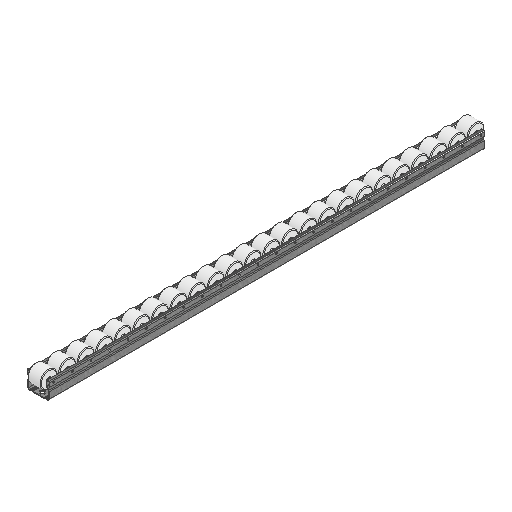
# Autodesk Inventor part: Trilho Roletado Flow Rack 40
Saved by Autodesk Inventor 2026.1 (Build 301233000, 233)
## iProperties
Company: Elgin
Created: 2024-05-28
Part Number: Trilho Roletado Flow Rack 40
Material: Genérico
Document SubType Name: Modeling
Designer: Willian Pinheiro
Density: 1 g/cm^3
Appearance: Padrão
Mass: 662.162 g
Surface Area: 3287.54 cm^2
Volume: 662.162 cm^3
Checked By: Antonio Lucas
Engr Approved By: Antonio Lucas
Description: Trilho Roletado Flow Rack 40
Mfg Approved By: Anderson Oliveira
Dimensões: 800 mm
Total: 8
Author: Willian Pinheiro
Title: Ceteva
Revision Number: 00
Autodesk Inventor part; units mm, degrees
ref_plane "YZ Plane" through (0, 0, 0) normal (1, 0, 0) x (0, 1, 0)
sketch "trilho roletado 40" plane through (0, 0, 0) normal (0, 0, 1) x (1, 0, 0)
  line L0 (54.5, 1.2) -> (54.5, -1.2)
  line L1 (54.5, -1.2) -> (54, -1.7)
  line L2 (54, -1.7) -> (16, -1.7)
  line L3 (49, -1.7) -> (49, -4)
  line L4 (49, -4) -> (47.5, -4)
  line L5 (47.5, -4) -> (47.5, -14.6092)
  arc A0 (46.1065, -16.1054) -> (47.5, -14.6092) centre (46, -14.6092) ccw
  arc A1 (23.8935, -16.1054) -> (46.1065, -16.1054) centre (35, 140) ccw
  arc A2 (22.5, -14.6092) -> (23.8935, -16.1054) centre (24, -14.6092) ccw
  line L6 (22.5, -14.6092) -> (22.5, -4)
  line L7 (22.5, -4) -> (21, -4)
  line L8 (21, -4) -> (21, -1.7)
  line L9 (16, -1.7) -> (15.5, -1.2)
  line L10 (15.5, -1.2) -> (15.5, 1.2)
  line L11 (15.5, 1.2) -> (16, 1.7)
  line L12 (21, 1.7) -> (21, 4)
  line L13 (21, 4) -> (22.5, 4)
  line L14 (22.5, 4) -> (22.5, 14.6092)
  arc A3 (23.8935, 16.1054) -> (22.5, 14.6092) centre (24, 14.6092) ccw
  arc A4 (46.1065, 16.1054) -> (23.8935, 16.1054) centre (35, -140) ccw
  arc A5 (47.5, 14.6092) -> (46.1065, 16.1054) centre (46, 14.6092) ccw
  line L15 (47.5, 14.6092) -> (47.5, 4)
  line L16 (47.5, 4) -> (49, 4)
  line L17 (49, 4) -> (49, 1.7)
  line L18 (16, 1.7) -> (54, 1.7)
  line L19 (54, 1.7) -> (54.5, 1.2)
  line L20 (13.5, -1.7865) -> (15, -1.7865)
  line L21 (15, -1.7865) -> (15, -4.5365)
  line L22 (15, -4.5365) -> (13.5, -4.5365)
  line L23 (13.5, -4.5365) -> (13.5, -1.7865)
  line L24 (20.5, 1.7135) -> (19, 1.7135)
  line L25 (19, 1.7135) -> (19, 3)
  line L26 (19, 3) -> (15, 3)
  line L27 (15, 3) -> (15, 1.7135)
  line L28 (15, 1.7135) -> (13.5, 1.7135)
  line L29 (13.5, 1.7135) -> (13.5, 3)
  arc A6 (15, 4.5) -> (13.5, 3) centre (15, 3) ccw
  line L30 (15, 4.5) -> (19, 4.5)
  arc A7 (20.5, 3) -> (19, 4.5) centre (19, 3) ccw
  line L31 (20.5, 3) -> (20.5, 1.7135)
  line L32 (56.5, 1.7135) -> (55, 1.7135)
  line L33 (55, 1.7135) -> (55, 3)
  line L34 (55, 3) -> (51, 3)
  line L35 (51, 3) -> (51, 1.7135)
  line L36 (51, 1.7135) -> (49.5, 1.7135)
  line L37 (49.5, 1.7135) -> (49.5, 3)
  arc A8 (51, 4.5) -> (49.5, 3) centre (51, 3) ccw
  line L38 (51, 4.5) -> (55, 4.5)
  arc A9 (56.5, 3) -> (55, 4.5) centre (55, 3) ccw
  line L39 (56.5, 3) -> (56.5, 1.7135)
  line L40 (55, -1.7865) -> (56.5, -1.7865)
  line L41 (56.5, -1.7865) -> (56.5, -4.5365)
  line L42 (56.5, -4.5365) -> (55, -4.5365)
  line L43 (55, -4.5365) -> (55, -1.7865)
  line L44 (40.75, -27) -> (45.3477, -27)
  arc A10 (45.3477, -27) -> (46.2081, -26.7287) centre (45.3477, -25.5) ccw
  line L45 (46.2081, -26.7287) -> (47.283, -25.9761)
  arc A11 (48.717, -25.9761) -> (47.283, -25.9761) centre (48, -27) ccw
  line L46 (48.717, -25.9761) -> (49.7919, -26.7287)
  arc A12 (49.7919, -26.7287) -> (50.6523, -27) centre (50.6523, -25.5) ccw
  line L47 (50.6523, -27) -> (51.5, -27)
  arc A13 (51.5, -27) -> (53.5, -25) centre (51.5, -25) ccw
  line L48 (53.5, -25) -> (53.5, -12.7967)
  arc A14 (53.5, -12.7967) -> (53.1047, -11.3083) centre (50.5, -12.7967) ccw
  line L49 (53.1047, -11.3083) -> (49.8953, -5.6917)
  arc A15 (49.5, -4.1668) -> (49.8953, -5.6917) centre (52.4998, -4.2029) ccw
  line L50 (49.5, -4.1668) -> (49.5, -1.7135)
  line L51 (49.5, -1.7135) -> (51, -1.7135)
  line L52 (51, -1.7135) -> (51, -4.1668)
  arc A16 (51, -4.1668) -> (51.1976, -4.9475) centre (52.4996, -4.2026) ccw
  line L53 (51.1976, -4.9475) -> (54.4071, -10.5641)
  arc A17 (55, -12.7967) -> (54.4071, -10.5641) centre (50.5, -12.7967) ccw
  line L54 (55, -12.7967) -> (55, -25)
  arc A18 (51.5, -28.5) -> (55, -25) centre (51.5, -25) ccw
  line L55 (51.5, -28.5) -> (50.6523, -28.5)
  arc A19 (48.9315, -27.9575) -> (50.6523, -28.5) centre (50.6523, -25.5) ccw
  line L56 (48.9315, -27.9575) -> (48, -27.3052)
  line L57 (48, -27.3052) -> (47.0685, -27.9575)
  arc A20 (45.3477, -28.5) -> (47.0685, -27.9575) centre (45.3477, -25.5) ccw
  line L58 (45.3477, -28.5) -> (40.75, -28.5)
  line L59 (29.25, -28.5) -> (24.6523, -28.5)
  arc A21 (22.9315, -27.9575) -> (24.6523, -28.5) centre (24.6523, -25.5) ccw
  line L60 (22.9315, -27.9575) -> (22, -27.3052)
  line L61 (22, -27.3052) -> (21.0685, -27.9575)
  arc A22 (19.3477, -28.5) -> (21.0685, -27.9575) centre (19.3477, -25.5) ccw
  line L62 (19.3477, -28.5) -> (18.5, -28.5)
  arc A23 (15, -25) -> (18.5, -28.5) centre (18.5, -25) ccw
  line L63 (15, -25) -> (15, -12.7967)
  arc A24 (15.5929, -10.5276) -> (15, -12.7967) centre (19.4999, -12.7605) ccw
  line L64 (15.5929, -10.5276) -> (18.8024, -4.911)
  arc A25 (18.8024, -4.911) -> (19, -4.1668) centre (17.5, -4.1668) ccw
  line L65 (19, -4.1668) -> (19, -1.7135)
  line L66 (19, -1.7135) -> (20.5, -1.7135)
  line L67 (20.5, -1.7135) -> (20.5, -4.2398)
  arc A26 (20.1047, -5.7282) -> (20.5, -4.2398) centre (17.5, -4.2398) ccw
  line L68 (20.1047, -5.7282) -> (16.8953, -11.3448)
  arc A27 (16.8953, -11.3448) -> (16.5, -12.7967) centre (19.4998, -12.8336) ccw
  line L69 (16.5, -12.7967) -> (16.5, -25)
  arc A28 (16.5, -25) -> (18.5, -27) centre (18.5, -25) ccw
  line L70 (18.5, -27) -> (19.3477, -27)
  arc A29 (19.3477, -27) -> (20.2081, -26.7287) centre (19.3477, -25.5) ccw
  line L71 (20.2081, -26.7287) -> (21.283, -25.9761)
  arc A30 (22.717, -25.9761) -> (21.283, -25.9761) centre (22, -27) ccw
  line L72 (22.717, -25.9761) -> (23.7919, -26.7287)
  arc A31 (23.7919, -26.7287) -> (24.6523, -27) centre (24.6523, -25.5) ccw
  line L73 (24.6523, -27) -> (29.25, -27)
  line L74 (29.25, -27) -> (29.25, -28.5)
  line L75 (40.75, -27) -> (40.75, -28.5)
  line L76 (29.25, -27) -> (40.75, -27)
  line L77 (40.75, -28.5) -> (29.25, -28.5)
  line L78 (13.5, 1.7135) -> (13.5, -1.7865)
  line L79 (15, 1.7135) -> (15, -1.7865)
  line L80 (19, 1.7135) -> (19, -1.7135)
  line L81 (20.5, -1.7135) -> (20.5, 1.7135)
  line L82 (49.5, 1.7135) -> (49.5, -1.7135)
  line L83 (51, 1.7135) -> (51, -1.7135)
  line L84 (55, 1.7135) -> (55, -1.7865)
  line L85 (56.5, 1.7135) -> (56.5, -1.7865)
  line L86 (35, -28.5) -> (35, -27) construction
  line L87 (54.5, 0) -> (15.5, 0)
  point P0 (35, 0)
  dimension "d40" = 1.5
  dimension "d41" = 1.5
  dimension "d42" = 33
  dimension "d43" = 1.5
  dimension "d44" = 1.5
  dimension "d45" = 1.5
  measures "d40" distance between parallel lines of L26 L30
  measures "d41" radius of A6
  measures "d42" distance between parallel lines of L59 L30
  measures "d43" distance between parallel lines of L27 L29
  measures "d44" distance between parallel lines of L31 L25
  measures "d45" distance between parallel lines of L59 L73
sketch "Sketch1" plane through (0, 0, 0) normal (0, 1, 0) x (-1, 0, 0)
  line L0 (30.5349, 0) -> (-30.5349, 0) construction
  line L1 (0, -167.5) -> (0, 224.5) construction
  line L2 (19.5, 29.7) -> (19.5, 27.3)
  line L3 (19.5, 27.3) -> (19, 26.8)
  line L4 (19, 26.8) -> (-19, 26.8)
  line L5 (14, 26.8) -> (14, 24.5)
  line L6 (14, 24.5) -> (12.5, 24.5)
  line L7 (12.5, 24.5) -> (12.5, 13.8908)
  arc A0 (11.1065, 12.3946) -> (12.5, 13.8908) centre (11, 13.8908) ccw
  arc A1 (-11.1065, 12.3946) -> (11.1065, 12.3946) centre (0, 168.5) ccw
  arc A2 (-12.5, 13.8908) -> (-11.1065, 12.3946) centre (-11, 13.8908) ccw
  line L8 (-12.5, 13.8908) -> (-12.5, 24.5)
  line L9 (-12.5, 24.5) -> (-14, 24.5)
  line L10 (-14, 24.5) -> (-14, 26.8)
  line L11 (-19, 26.8) -> (-19.5, 27.3)
  line L12 (-19.5, 27.3) -> (-19.5, 29.7)
  line L13 (-19.5, 29.7) -> (-19, 30.2)
  line L14 (-14, 30.2) -> (-14, 32.5)
  line L15 (-14, 32.5) -> (-12.5, 32.5)
  line L16 (-12.5, 32.5) -> (-12.5, 43.1092)
  arc A3 (-11.1065, 44.6054) -> (-12.5, 43.1092) centre (-11, 43.1092) ccw
  arc A4 (11.1065, 44.6054) -> (-11.1065, 44.6054) centre (0, -111.5) ccw
  arc A5 (12.5, 43.1092) -> (11.1065, 44.6054) centre (11, 43.1092) ccw
  line L17 (12.5, 43.1092) -> (12.5, 32.5)
  line L18 (12.5, 32.5) -> (14, 32.5)
  line L19 (14, 32.5) -> (14, 30.2)
  line L20 (-19, 30.2) -> (19, 30.2)
  line L21 (19, 30.2) -> (19.5, 29.7)
  line L22 (-21.5, 26.7135) -> (-20, 26.7135)
  line L23 (-20, 26.7135) -> (-20, 23.9635)
  line L24 (-20, 23.9635) -> (-21.5, 23.9635)
  line L25 (-21.5, 23.9635) -> (-21.5, 26.7135)
  line L26 (-14.5, 30.2135) -> (-16, 30.2135)
  line L27 (-16, 30.2135) -> (-16, 31.5)
  line L28 (-16, 31.5) -> (-20, 31.5)
  line L29 (-20, 31.5) -> (-20, 30.2135)
  line L30 (-20, 30.2135) -> (-21.5, 30.2135)
  line L31 (-21.5, 30.2135) -> (-21.5, 31.5)
  arc A6 (-20, 33) -> (-21.5, 31.5) centre (-20, 31.5) ccw
  line L32 (-20, 33) -> (-16, 33)
  arc A7 (-14.5, 31.5) -> (-16, 33) centre (-16, 31.5) ccw
  line L33 (-14.5, 31.5) -> (-14.5, 30.2135)
  line L34 (21.5, 30.2135) -> (20, 30.2135)
  line L35 (20, 30.2135) -> (20, 31.5)
  line L36 (20, 31.5) -> (16, 31.5)
  line L37 (16, 31.5) -> (16, 30.2135)
  line L38 (16, 30.2135) -> (14.5, 30.2135)
  line L39 (14.5, 30.2135) -> (14.5, 31.5)
  arc A8 (16, 33) -> (14.5, 31.5) centre (16, 31.5) ccw
  line L40 (16, 33) -> (20, 33)
  arc A9 (21.5, 31.5) -> (20, 33) centre (20, 31.5) ccw
  line L41 (21.5, 31.5) -> (21.5, 30.2135)
  line L42 (20, 26.7135) -> (21.5, 26.7135)
  line L43 (21.5, 26.7135) -> (21.5, 23.9635)
  line L44 (21.5, 23.9635) -> (20, 23.9635)
  line L45 (20, 23.9635) -> (20, 26.7135)
  line L46 (5.75, 1.5) -> (10.3477, 1.5)
  arc A10 (10.3477, 1.5) -> (11.2081, 1.7713) centre (10.3477, 3) ccw
  line L47 (11.2081, 1.7713) -> (12.283, 2.5239)
  arc A11 (13.717, 2.5239) -> (12.283, 2.5239) centre (13, 1.5) ccw
  line L48 (13.717, 2.5239) -> (14.7919, 1.7713)
  arc A12 (14.7919, 1.7713) -> (15.6523, 1.5) centre (15.6523, 3) ccw
  line L49 (15.6523, 1.5) -> (16.5, 1.5)
  arc A13 (16.5, 1.5) -> (18.5, 3.5) centre (16.5, 3.5) ccw
  line L50 (18.5, 3.5) -> (18.5, 15.7033)
  arc A14 (18.5, 15.7033) -> (18.1047, 17.1917) centre (15.5, 15.7033) ccw
  line L51 (18.1047, 17.1917) -> (14.8953, 22.8083)
  arc A15 (14.5, 24.3332) -> (14.8953, 22.8083) centre (17.4998, 24.2971) ccw
  line L52 (14.5, 24.3332) -> (14.5, 26.7865)
  line L53 (14.5, 26.7865) -> (16, 26.7865)
  line L54 (16, 26.7865) -> (16, 24.3332)
  arc A16 (16, 24.3332) -> (16.1976, 23.5525) centre (17.4996, 24.2974) ccw
  line L55 (16.1976, 23.5525) -> (19.4071, 17.9359)
  arc A17 (20, 15.7033) -> (19.4071, 17.9359) centre (15.5, 15.7033) ccw
  line L56 (20, 15.7033) -> (20, 3.5)
  arc A18 (16.5, 0) -> (20, 3.5) centre (16.5, 3.5) ccw
  line L57 (16.5, 0) -> (15.6523, 0)
  arc A19 (13.9315, 0.5425) -> (15.6523, 0) centre (15.6523, 3) ccw
  line L58 (13.9315, 0.5425) -> (13, 1.1948)
  line L59 (13, 1.1948) -> (12.0685, 0.5425)
  arc A20 (10.3477, 0) -> (12.0685, 0.5425) centre (10.3477, 3) ccw
  line L60 (10.3477, 0) -> (5.75, 0)
  line L61 (-5.75, 0) -> (-10.3477, 0)
  arc A21 (-12.0685, 0.5425) -> (-10.3477, 0) centre (-10.3477, 3) ccw
  line L62 (-12.0685, 0.5425) -> (-13, 1.1948)
  line L63 (-13, 1.1948) -> (-13.9315, 0.5425)
  arc A22 (-15.6523, 0) -> (-13.9315, 0.5425) centre (-15.6523, 3) ccw
  line L64 (-15.6523, 0) -> (-16.5, 0)
  arc A23 (-20, 3.5) -> (-16.5, 0) centre (-16.5, 3.5) ccw
  line L65 (-20, 3.5) -> (-20, 15.7033)
  arc A24 (-19.4071, 17.9724) -> (-20, 15.7033) centre (-15.5001, 15.7395) ccw
  line L66 (-19.4071, 17.9724) -> (-16.1976, 23.589)
  arc A25 (-16.1976, 23.589) -> (-16, 24.3332) centre (-17.5, 24.3332) ccw
  line L67 (-16, 24.3332) -> (-16, 26.7865)
  line L68 (-16, 26.7865) -> (-14.5, 26.7865)
  line L69 (-14.5, 26.7865) -> (-14.5, 24.2602)
  arc A26 (-14.8953, 22.7718) -> (-14.5, 24.2602) centre (-17.5, 24.2602) ccw
  line L70 (-14.8953, 22.7718) -> (-18.1047, 17.1552)
  arc A27 (-18.1047, 17.1552) -> (-18.5, 15.7033) centre (-15.5002, 15.6664) ccw
  line L71 (-18.5, 15.7033) -> (-18.5, 3.5)
  arc A28 (-18.5, 3.5) -> (-16.5, 1.5) centre (-16.5, 3.5) ccw
  line L72 (-16.5, 1.5) -> (-15.6523, 1.5)
  arc A29 (-15.6523, 1.5) -> (-14.7919, 1.7713) centre (-15.6523, 3) ccw
  line L73 (-14.7919, 1.7713) -> (-13.717, 2.5239)
  arc A30 (-12.283, 2.5239) -> (-13.717, 2.5239) centre (-13, 1.5) ccw
  line L74 (-12.283, 2.5239) -> (-11.2081, 1.7713)
  arc A31 (-11.2081, 1.7713) -> (-10.3477, 1.5) centre (-10.3477, 3) ccw
  line L75 (-10.3477, 1.5) -> (-5.75, 1.5)
  line L76 (-5.75, 1.5) -> (-5.75, 0)
  line L77 (5.75, 1.5) -> (5.75, 0)
  line L78 (-5.75, 1.5) -> (5.75, 1.5)
  line L79 (5.75, 0) -> (-5.75, 0)
  line L80 (-21.5, 30.2135) -> (-21.5, 26.7135)
  line L81 (-20, 30.2135) -> (-20, 26.7135)
  line L82 (-16, 30.2135) -> (-16, 26.7865)
  line L83 (-14.5, 26.7865) -> (-14.5, 30.2135)
  line L84 (14.5, 30.2135) -> (14.5, 26.7865)
  line L85 (16, 30.2135) -> (16, 26.7865)
  line L86 (20, 30.2135) -> (20, 26.7135)
  line L87 (21.5, 30.2135) -> (21.5, 26.7135)
  line L88 (0, 0) -> (0, 1.5) construction
  line L89 (19.5, 28.5) -> (-19.5, 28.5)
  point P0 (0, 0)
  constraints: 1 horizontal, 1 vertical
extrude "Extrusion1" add sketch "Sketch1" along normal blind 820 contours L89 L84 L20 L85 | L85 L4 L84 L89 | L20 L84 L38 L85 | L85 L53 L84 L4 | L38 L39 A8 L40 A9 L41 L34 L35 L36 L37 | L54 A16 L55 A17 L56 A18 L57 A19 L58 L59 A20 L60 L77 L46 A10 L47 A11 L48 A12 L49 A13 L50 A14 L51 A15 L52 L53 | L89 L82 L20 L83 | L83 L4 L82 L89 | L83 L68 L82 L4 | L20 L82 L26 L83 | L69 A26 L70 A27 L71 A28 L72 A29 L73 A30 L74 A31 L75 L76 L61 A21 L62 L63 A22 L64 A23 L65 A24 L66 A25 L67 L68 | L26 L27 L28 L29 L30 L31 A6 L32 A7 L33 | L34 L87 L42 L86 | L42 L43 L44 L45 | L81 L22 L80 L30 | L23 L24 L25 L22 | L79 L76 L78 L77
sketch "Sketch2" plane through (0, -500, 24) normal (1, 0, 0) x (0, 0, -1)
  circle A0 centre (-4.5, 507.5) radius 1.75 construction
  line L0 (24, -198.35) -> (24, 1190.1) construction
  line L1 (30.3, 500) -> (-13.8, 500) construction
  circle A1 centre (-4.5, 542.5) radius 1.75 construction
  circle A2 centre (-4.5, 577.5) radius 1.75 construction
  circle A3 centre (-4.5, 612.5) radius 1.75 construction
  circle A4 centre (-4.5, 647.5) radius 1.75 construction
  circle A5 centre (-4.5, 682.5) radius 1.75 construction
  circle A6 centre (-4.5, 717.5) radius 1.75 construction
  circle A7 centre (-4.5, 752.5) radius 1.75 construction
  circle A8 centre (-4.5, 787.5) radius 1.75 construction
  circle A9 centre (-4.5, 822.5) radius 1.75 construction
  circle A10 centre (-4.5, 857.5) radius 1.75 construction
  circle A11 centre (-4.5, 892.5) radius 1.75 construction
  circle A12 centre (-4.5, 927.5) radius 1.75 construction
  circle A13 centre (-4.5, 962.5) radius 1.75 construction
  circle A14 centre (-4.5, 997.5) radius 1.75 construction
  circle A15 centre (-4.5, 1032.5) radius 1.75 construction
  circle A16 centre (-4.5, 1067.5) radius 1.75 construction
  circle A17 centre (-4.5, 1102.5) radius 1.75 construction
  circle A18 centre (-4.5, 1137.5) radius 1.75 construction
  circle A19 centre (-4.5, 1172.5) radius 1.75 construction
  circle A20 centre (-4.5, 1207.5) radius 1.75 construction
  circle A21 centre (-4.5, 1242.5) radius 1.75 construction
  circle A22 centre (-4.5, 1277.5) radius 1.75 construction
  line L2 (-7.5, 1320) -> (-0.3332, 1320) projected
  circle A23 centre (-4.5, 1312.5) radius 1.75 construction
  point P0 (24, 500)
  dimension "d3" = 3.5
  dimension "d6" = 35
  dimension "d13" = 7.5
  dimension "d14" = 820
  constraints: 24 centre point, 2 end point, 1 vertical, 46 other
  measures "d3" diameter of A0
  measures "d6" distance of A0.centre A1.centre
  measures "d13" distance from line of A0.centre L1
  measures "d14" distance between parallel lines of L2 L1
hole "Hole1" at (0, 7.5, 28.5) direction (-1, 0, 0) diameter 3.5 end through all both
ref_plane "Work Plane1" through (0, 7.5, 28.5) normal (0, -1, 0) x (1, 0, 0)
sketch "Sketch4" plane through (-10.3477, 0, 1.5) normal (0, 0, 1) x (1, 0, 0)
  line L0 (40.4477, 7.5) -> (-19.7523, 7.5) construction
  line L1 (10.3477, -164) -> (10.3477, 984) construction
  arc A0 (11.5803, 12.2084) -> (9.1152, 12.2084) centre (10.3477, 12) ccw
  arc A1 (5.6394, 8.7325) -> (5.6394, 6.2675) centre (5.8477, 7.5) ccw
  arc A2 (15.0561, 6.2675) -> (15.0561, 8.7325) centre (14.8477, 7.5) ccw
  arc A3 (9.1152, 2.7916) -> (11.5803, 2.7916) centre (10.3477, 3) ccw
  line L2 (9.1152, 2.7916) -> (8.7903, 4.7136)
  line L3 (11.5803, 2.7916) -> (11.9052, 4.7136)
  line L4 (9.1152, 12.2084) -> (8.7903, 10.2864)
  line L5 (5.6394, 6.2675) -> (7.5613, 5.9426)
  line L6 (5.6394, 8.7325) -> (7.5613, 9.0574)
  line L7 (15.0561, 6.2675) -> (13.1341, 5.9426)
  arc A4 (8.7903, 4.7136) -> (7.5613, 5.9426) centre (7.3113, 4.4636) ccw
  arc A5 (7.5613, 9.0574) -> (8.7903, 10.2864) centre (7.3113, 10.5364) ccw
  arc A6 (13.1341, 5.9426) -> (11.9052, 4.7136) centre (13.3842, 4.4636) ccw
  arc A7 (11.9052, 10.2864) -> (13.1341, 9.0574) centre (13.3842, 10.5364) ccw
  line L8 (11.5803, 12.2084) -> (11.9052, 10.2864)
  line L9 (12.0829, 14.2351) -> (12.0829, 14.2348)
  line L10 (15.0561, 8.7325) -> (13.1341, 9.0574)
  line L11 (12.0829, 14.2351) -> (12.0826, 14.2352)
  point P0 (10.3477, 0)
  point P1 (12.0829, 0.7652)
  point P2 (8.6129, 14.2352)
  dimension "d28" = 2.5
  dimension "d29" = 9
  dimension "d30" = 9
  dimension "d31" = 19.19
  dimension "d32" = 19.19
  dimension "d33" = 3
  constraints: 20 end point, 16 point on circle, 13 symmetric about line, 8 centre point, 4 tangent, 2 point on line, 1 equal radius, 7 other
  measures "d28" diameter of A0
  measures "d29" distance of A3.centre A0.centre
  measures "d30" distance of A2.centre A1.centre
  measures "d31" angle of L3 L2
  measures "d32" angle of L6 L5
  measures "d33" diameter of A4
extrude "Extrusion2" cut sketch "Sketch4" along normal through all both and the other way through all
sketch "Sketch3" plane through (0, 7.5, 28.5) normal (0, -1, 0) x (1, 0, 0)
  line L0 (-30.5349, -28.5) -> (30.5349, -28.5) construction
  line L1 (0, -196) -> (0, 196) construction
  line L2 (10.3477, -28.5) -> (-10.3477, -28.5) projected
  line L3 (19.5, 1.2) -> (19.5, -1.2)
  line L4 (19.5, -1.2) -> (19, -1.7)
  line L5 (19, -1.7) -> (-19, -1.7)
  line L6 (14, -1.7) -> (14, -4)
  line L7 (14, -4) -> (12.5, -4)
  line L8 (12.5, -4) -> (12.5, -14.6092)
  arc A0 (11.1065, -16.1054) -> (12.5, -14.6092) centre (11, -14.6092) ccw
  arc A1 (-11.1065, -16.1054) -> (11.1065, -16.1054) centre (0, 140) ccw
  arc A2 (-12.5, -14.6092) -> (-11.1065, -16.1054) centre (-11, -14.6092) ccw
  line L9 (-12.5, -14.6092) -> (-12.5, -4)
  line L10 (-12.5, -4) -> (-14, -4)
  line L11 (-14, -4) -> (-14, -1.7)
  line L12 (-19, -1.7) -> (-19.5, -1.2)
  line L13 (-19.5, -1.2) -> (-19.5, 1.2)
  line L14 (-19.5, 1.2) -> (-19, 1.7)
  line L15 (-14, 1.7) -> (-14, 4)
  line L16 (-14, 4) -> (-12.5, 4)
  line L17 (-12.5, 4) -> (-12.5, 14.6092)
  arc A3 (-11.1065, 16.1054) -> (-12.5, 14.6092) centre (-11, 14.6092) ccw
  arc A4 (11.1065, 16.1054) -> (-11.1065, 16.1054) centre (0, -140) ccw
  arc A5 (12.5, 14.6092) -> (11.1065, 16.1054) centre (11, 14.6092) ccw
  line L18 (12.5, 14.6092) -> (12.5, 4)
  line L19 (12.5, 4) -> (14, 4)
  line L20 (14, 4) -> (14, 1.7)
  line L21 (-19, 1.7) -> (19, 1.7)
  line L22 (19, 1.7) -> (19.5, 1.2)
  line L23 (-21.5, -1.7865) -> (-20, -1.7865)
  line L24 (-20, -1.7865) -> (-20, -4.5365)
  line L25 (-20, -4.5365) -> (-21.5, -4.5365)
  line L26 (-21.5, -4.5365) -> (-21.5, -1.7865)
  line L27 (-14.5, 1.7135) -> (-16, 1.7135)
  line L28 (-16, 1.7135) -> (-16, 3)
  line L29 (-16, 3) -> (-20, 3)
  line L30 (-20, 3) -> (-20, 1.7135)
  line L31 (-20, 1.7135) -> (-21.5, 1.7135)
  line L32 (-21.5, 1.7135) -> (-21.5, 3)
  arc A6 (-20, 4.5) -> (-21.5, 3) centre (-20, 3) ccw
  line L33 (-20, 4.5) -> (-16, 4.5)
  arc A7 (-14.5, 3) -> (-16, 4.5) centre (-16, 3) ccw
  line L34 (-14.5, 3) -> (-14.5, 1.7135)
  line L35 (21.5, 1.7135) -> (20, 1.7135)
  line L36 (20, 1.7135) -> (20, 3)
  line L37 (20, 3) -> (16, 3)
  line L38 (16, 3) -> (16, 1.7135)
  line L39 (16, 1.7135) -> (14.5, 1.7135)
  line L40 (14.5, 1.7135) -> (14.5, 3)
  arc A8 (16, 4.5) -> (14.5, 3) centre (16, 3) ccw
  line L41 (16, 4.5) -> (20, 4.5)
  arc A9 (21.5, 3) -> (20, 4.5) centre (20, 3) ccw
  line L42 (21.5, 3) -> (21.5, 1.7135)
  line L43 (20, -1.7865) -> (21.5, -1.7865)
  line L44 (21.5, -1.7865) -> (21.5, -4.5365)
  line L45 (21.5, -4.5365) -> (20, -4.5365)
  line L46 (20, -4.5365) -> (20, -1.7865)
  line L47 (5.75, -27) -> (10.3477, -27)
  arc A10 (10.3477, -27) -> (11.2081, -26.7287) centre (10.3477, -25.5) ccw
  line L48 (11.2081, -26.7287) -> (12.283, -25.9761)
  arc A11 (13.717, -25.9761) -> (12.283, -25.9761) centre (13, -27) ccw
  line L49 (13.717, -25.9761) -> (14.7919, -26.7287)
  arc A12 (14.7919, -26.7287) -> (15.6523, -27) centre (15.6523, -25.5) ccw
  line L50 (15.6523, -27) -> (16.5, -27)
  arc A13 (16.5, -27) -> (18.5, -25) centre (16.5, -25) ccw
  line L51 (18.5, -25) -> (18.5, -12.7967)
  arc A14 (18.5, -12.7967) -> (18.1047, -11.3083) centre (15.5, -12.7967) ccw
  line L52 (18.1047, -11.3083) -> (14.8953, -5.6917)
  arc A15 (14.5, -4.1668) -> (14.8953, -5.6917) centre (17.4998, -4.2029) ccw
  line L53 (14.5, -4.1668) -> (14.5, -1.7135)
  line L54 (14.5, -1.7135) -> (16, -1.7135)
  line L55 (16, -1.7135) -> (16, -4.1668)
  arc A16 (16, -4.1668) -> (16.1976, -4.9475) centre (17.4996, -4.2026) ccw
  line L56 (16.1976, -4.9475) -> (19.4071, -10.5641)
  arc A17 (20, -12.7967) -> (19.4071, -10.5641) centre (15.5, -12.7967) ccw
  line L57 (20, -12.7967) -> (20, -25)
  arc A18 (16.5, -28.5) -> (20, -25) centre (16.5, -25) ccw
  line L58 (16.5, -28.5) -> (15.6523, -28.5)
  arc A19 (13.9315, -27.9575) -> (15.6523, -28.5) centre (15.6523, -25.5) ccw
  line L59 (13.9315, -27.9575) -> (13, -27.3052)
  line L60 (13, -27.3052) -> (12.0685, -27.9575)
  arc A20 (10.3477, -28.5) -> (12.0685, -27.9575) centre (10.3477, -25.5) ccw
  line L61 (10.3477, -28.5) -> (5.75, -28.5)
  line L62 (-5.75, -28.5) -> (-10.3477, -28.5)
  arc A21 (-12.0685, -27.9575) -> (-10.3477, -28.5) centre (-10.3477, -25.5) ccw
  line L63 (-12.0685, -27.9575) -> (-13, -27.3052)
  line L64 (-13, -27.3052) -> (-13.9315, -27.9575)
  arc A22 (-15.6523, -28.5) -> (-13.9315, -27.9575) centre (-15.6523, -25.5) ccw
  line L65 (-15.6523, -28.5) -> (-16.5, -28.5)
  arc A23 (-20, -25) -> (-16.5, -28.5) centre (-16.5, -25) ccw
  line L66 (-20, -25) -> (-20, -12.7967)
  arc A24 (-19.4071, -10.5276) -> (-20, -12.7967) centre (-15.5001, -12.7605) ccw
  line L67 (-19.4071, -10.5276) -> (-16.1976, -4.911)
  arc A25 (-16.1976, -4.911) -> (-16, -4.1668) centre (-17.5, -4.1668) ccw
  line L68 (-16, -4.1668) -> (-16, -1.7135)
  line L69 (-16, -1.7135) -> (-14.5, -1.7135)
  line L70 (-14.5, -1.7135) -> (-14.5, -4.2398)
  arc A26 (-14.8953, -5.7282) -> (-14.5, -4.2398) centre (-17.5, -4.2398) ccw
  line L71 (-14.8953, -5.7282) -> (-18.1047, -11.3448)
  arc A27 (-18.1047, -11.3448) -> (-18.5, -12.7967) centre (-15.5002, -12.8336) ccw
  line L72 (-18.5, -12.7967) -> (-18.5, -25)
  arc A28 (-18.5, -25) -> (-16.5, -27) centre (-16.5, -25) ccw
  line L73 (-16.5, -27) -> (-15.6523, -27)
  arc A29 (-15.6523, -27) -> (-14.7919, -26.7287) centre (-15.6523, -25.5) ccw
  line L74 (-14.7919, -26.7287) -> (-13.717, -25.9761)
  arc A30 (-12.283, -25.9761) -> (-13.717, -25.9761) centre (-13, -27) ccw
  line L75 (-12.283, -25.9761) -> (-11.2081, -26.7287)
  arc A31 (-11.2081, -26.7287) -> (-10.3477, -27) centre (-10.3477, -25.5) ccw
  line L76 (-10.3477, -27) -> (-5.75, -27)
  line L77 (-5.75, -27) -> (-5.75, -28.5)
  line L78 (5.75, -27) -> (5.75, -28.5)
  line L79 (-5.75, -27) -> (5.75, -27)
  line L80 (5.75, -28.5) -> (-5.75, -28.5)
  line L81 (-21.5, 1.7135) -> (-21.5, -1.7865)
  line L82 (-20, 1.7135) -> (-20, -1.7865)
  line L83 (-16, 1.7135) -> (-16, -1.7135)
  line L84 (-14.5, -1.7135) -> (-14.5, 1.7135)
  line L85 (14.5, 1.7135) -> (14.5, -1.7135)
  line L86 (16, 1.7135) -> (16, -1.7135)
  line L87 (20, 1.7135) -> (20, -1.7865)
  line L88 (21.5, 1.7135) -> (21.5, -1.7865)
  line L89 (0, -28.5) -> (0, -27) construction
  line L90 (19.5, 0) -> (-19.5, 0)
  point P0 (0, -28.5)
  point P1 (0, -28.5)
  constraints: 1 horizontal, 1 midpoint, 1 other
revolve "Revolution1" add sketch "Sketch3" angle 360 about axis through (19.5, 7.5, 28.5) along (-1, 0, 0) separate body contours L90 L85 L21 L86 | L86 L21 L22 L3 L90 | L90 L84 L21 L85 | L90 L83 L21 L84 | L90 L13 L14 L21 L83
revolve "Revolution2" add sketch "Sketch3" angle 360 about axis through (19.5, 7.5, 28.5) along (-1, 0, 0) separate body contours L21 L15 L16 L17 A3 A4 A5 L18 L19 L20
pattern_linear "Rectangular Pattern1" count 24 spacing 35 along (0, 1, 0) of "Hole1", "Extrusion2" bodies 1
ref_plane "Work Plane2" through (0, 410, 0) normal (0, -1, 0) x (1, 0, 0)
pattern_linear "Rectangular Pattern2" count 24 spacing 35 along (0, 1, 0) bodies 2 3
equation "\"d30\" = d29"
equation "\"d32\" = d31"
equation "\"d24\" = d6"
equation "\"d38\" = d6"
body "Solid1"
body "Solid2"
body "Solid3"
